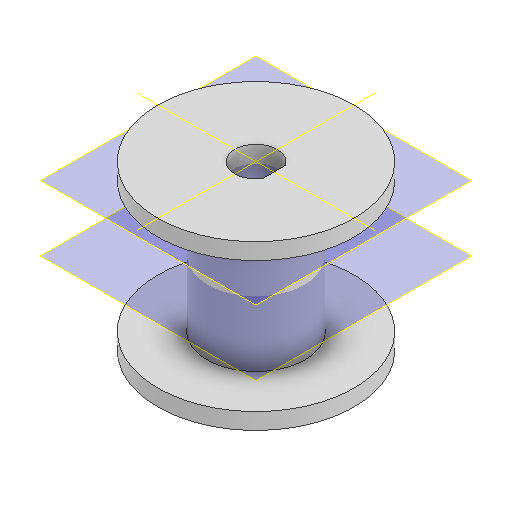
# Autodesk Inventor part: 도르래_new
Saved by Autodesk Inventor 2027 (Build 310192000, 192)
## iProperties
Created: 2026-09-17
Part Number: 도르래_new
Material: 일반
Document SubType Name: Modeling
Designer: User
Density: 1 g/cm^3
Appearance: 기본값
Author: User
Autodesk Inventor part; units mm, degrees
ref_plane "YZ 평면_우측면도" through (0, 0, 0) normal (1, 0, 0) x (0, 1, 0)
ref_plane "XZ 평면_평면도" through (0, 0, 0) normal (0, 1, 0) x (-1, 0, 0)
ref_plane "XY 평면_정면도" through (0, 0, 0) normal (0, 0, 1) x (1, 0, 0)
sketch "스케치1" plane through (0, 0, 0) normal (0, 1, 0) x (-1, 0, 0)
  circle A0 centre (0, 0) radius 30
  arc A1 (-5, -3.3166) -> (-5, 3.3166) centre (0, 0) ccw construction
  line L0 (0, 6) -> (0, -6) construction
  line L1 (-5, 3.3166) -> (-5, -3.3166) construction
  line L2 (-5.5, -3.4641) -> (-5.5, 3.4641)
  arc A2 (-5.5, -3.4641) -> (-5.5, 3.4641) centre (0, 0) ccw
  dimension "d0" = 60
  dimension "d1" = 12
  dimension "d2" = 5
  dimension "d3" = 0.5
  constraints: 6 end point, 5 point on circle, 3 centre point, 2 coincident, 1 midpoint, 1 parallel, 1 vertical, 1 other
  measures "d0" diameter of A0
  measures "d1" diameter of A1
  measures "d2" distance between parallel lines of L0 L1
  measures "d3" radial gap between concentric circles of A1 A2
extrude "돌출1" add sketch "스케치1" against normal blind 5
ref_plane "작업 평면1" through (0, -5, 0) normal (0, -1, 0) x (1, 0, 0)
sketch "스케치2" plane through (0, -5, 0) normal (0, -1, 0) x (1, 0, 0)
  line L0 (-42, 0) -> (42, 0) projected
  line L1 (0, -42) -> (0, 42) projected
  circle A0 centre (0, 0) radius 15
  arc A1 (5.5, 3.4641) -> (5.5, -3.4641) centre (0, 0) ccw projected
  line L2 (5.5, 3.4641) -> (5.5, -3.4641) projected
  dimension "d7" = 30
  constraints: 1 centre point, 1 coincident
  measures "d7" diameter of A0
extrude "돌출2" add sketch "스케치2" along normal blind 40 contours A0 L1 A1 L0 | L0 A1 L1 A0 | A0 L0 L2 A1 L1 | L1 A1 L2 L0 A0
ref_plane "작업 평면2" through (0, -25, 0) normal (0, -1, 0) x (1, 0, 0)
mirror "미러1" about plane through (0, -25, 0) normal (0, -1, 0) of "돌출1"
